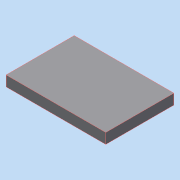
# Autodesk Inventor part: flat
Saved by Autodesk Inventor 2016 (Build 200138000, 138)
## iProperties
Created: 2017-03-05
Part Number: flat
Material: Generic
Document SubType Name: Modeling
Designer: Errrm
Density: 1 g/cm^3
Appearance: Default
Author: Errrm
Autodesk Inventor part; units mm, degrees
ref_plane "YZ Plane" through (0, 0, 0) normal (1, 0, 0) x (0, 1, 0)
ref_plane "XZ Plane" through (0, 0, 0) normal (0, 1, 0) x (-1, 0, 0)
ref_plane "XY Plane" through (0, 0, 0) normal (0, 0, 1) x (1, 0, 0)
sketch "Sketch1" plane through (0, 0, 0) normal (0, 0, 1) x (1, 0, 0)
  line L0 (-57.0182, 51.8235) -> (39.2078, 51.8235)
  line L1 (39.2078, 51.8235) -> (39.2078, -13.9763)
  line L2 (39.2078, -13.9763) -> (-57.0182, -13.9763)
  line L3 (-57.0182, -13.9763) -> (-57.0182, 51.8235)
  point P0 (0, 0)
  constraints: 8 end point, 2 parallel, 1 horizontal, 1 perpendicular
extrude "Extrusion1" add sketch "Sketch1" along normal blind 10
body "Solid1"
